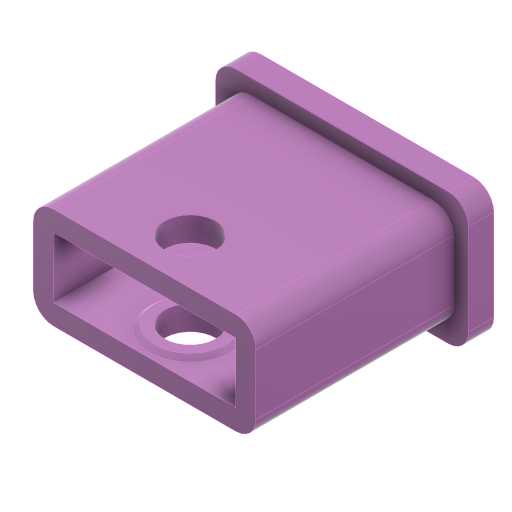
# Autodesk Inventor part: Короб для подшипника
Saved by Autodesk Inventor 2023 (Build 270158000, 158)
## iProperties
Created: 2023-02-25
Part Number: Короб для подшипника
Material: Типовые
Document SubType Name: Modeling
Designer: Admin
Density: 1 g/cm^3
Appearance: По умолчанию
Author: Admin
Autodesk Inventor part; units mm, degrees
ref_plane "YZ Plane" through (0, 0, 0) normal (1, 0, 0) x (0, 1, 0)
ref_plane "XZ Plane" through (0, 0, 0) normal (0, 1, 0) x (-1, 0, 0)
ref_plane "XY Plane" through (0, 0, 0) normal (0, 0, 1) x (1, 0, 0)
sketch "Эскиз1" plane through (0, 0, 0) normal (0, 0, 1) x (1, 0, 0)
  line L0 (-9, -5) -> (9, -5)
  line L1 (11, -3) -> (11, 3)
  line L2 (9, 5) -> (-9, 5)
  line L3 (-11, 3) -> (-11, -3)
  line L4 (-11, -5) -> (11, 5) construction
  line L5 (11, -5) -> (-11, 5) construction
  arc A0 (-9, 5) -> (-11, 3) centre (-9, 3) ccw
  arc A1 (-11, -3) -> (-9, -5) centre (-9, -3) ccw
  arc A2 (9, -5) -> (11, -3) centre (9, -3) ccw
  arc A3 (11, 3) -> (9, 5) centre (9, 3) ccw
  line L6 (-10.5, 6.5) -> (10.5, 6.5)
  line L7 (12.5, 4.5) -> (12.5, -4.5)
  line L8 (10.5, -6.5) -> (-10.5, -6.5)
  line L9 (-12.5, -4.5) -> (-12.5, 4.5)
  line L10 (-12.5, 6.5) -> (12.5, -6.5) construction
  line L11 (12.5, 6.5) -> (-12.5, -6.5) construction
  arc A4 (-10.5, 6.5) -> (-12.5, 4.5) centre (-10.5, 4.5) ccw
  arc A5 (-12.5, -4.5) -> (-10.5, -6.5) centre (-10.5, -4.5) ccw
  arc A6 (10.5, -6.5) -> (12.5, -4.5) centre (10.5, -4.5) ccw
  arc A7 (12.5, 4.5) -> (10.5, 6.5) centre (10.5, 4.5) ccw
  line L12 (-9, -3) -> (9, -3)
  line L13 (9, -3) -> (9, 3)
  line L14 (9, 3) -> (-9, 3)
  line L15 (-9, 3) -> (-9, -3)
  line L16 (-9, -3) -> (9, 3) construction
  line L17 (9, -3) -> (-9, 3) construction
  line L18 (0, 0) -> (7.9203, 0) construction
  dimension "Down_fit_y" = 10
  dimension "Down_fit_x" = 22
  dimension "d2" = 2
  dimension "Up_fit" = 1.5
  dimension "d4" = 1.5
  dimension "d5" = 2
  constraints: 38 end point, 16 point on circle, 16 point on line, 16 tangent, 8 centre point, 7 parallel, 6 equal radius, 6 midpoint, 3 horizontal, 3 perpendicular
  measures "Down_fit_y" distance between parallel lines of L0 L2
  measures "Down_fit_x" distance between parallel lines of L3 L1
  measures "d2" radius of A0
  measures "Up_fit" distance between parallel lines of L6 L2
  measures "d4" distance between parallel lines of L7 L1
  measures "d5" radius of A4
extrude "Выдавливание1" add sketch "Эскиз1" against normal blind 2.5 contours A1 L3 A0 L2 A3 L1 A2 L0 | L6 A7 L7 A6 L8 A5 L9 A4 | L15 L14 L13 L12
extrude "Выдавливание2" add sketch "Эскиз1" along normal blind 19.5 contours A1 L3 A0 L2 A3 L1 A2 L0
sketch "Эскиз2" plane through (-9, 5, 0) normal (0, 1, 0) x (1, 0, 0)
  circle A0 centre (9, -15) radius 2.5
  line L0 (6.6906, -11) -> (11.3094, -11)
  line L1 (11.3094, -11) -> (13.6188, -15)
  line L2 (13.6188, -15) -> (11.3094, -19)
  line L3 (11.3094, -19) -> (6.6906, -19)
  line L4 (6.6906, -19) -> (4.3812, -15)
  line L5 (4.3812, -15) -> (6.6906, -11)
  line L6 (-1.5, 2.5) -> (19.5, 2.5) projected
  line L7 (-2, 0) -> (-2, -19.5) projected
  line L8 (-2, -7.5) -> (20, -7.5) construction
  line L9 (20, 0) -> (20, -19.5) projected
  line L10 (19.5, 0) -> (-1.5, 0) projected
  circle A1 centre (9, -15) radius 8 construction
  line L11 (18, -19.5) -> (0, -19.5) projected
  point P0 (9, 0)
  point P1 (9, 0)
  dimension "hole" = 5
  dimension "d13" = 10
  dimension "d14" = 8
  dimension "d15" = 16
  dimension "d16" = 3.5
  constraints: 14 end point, 2 centre point, 2 coincident, 2 horizontal, 2 point on line, 1 midpoint, 1 vertical alignment, 13 other
  measures "hole" diameter of A0
  measures "d13" distance between parallel lines of L6 L8
  measures "d14" distance between parallel lines of L3 L0
  measures "d15" diameter of A1
  measures "d16" distance edge to line of A1 L11
extrude "Выдавливание3" cut sketch "Эскиз2" against normal through all contours A0
sketch "Эскиз3" plane through (-9, 3, 0) normal (0, -1, 0) x (1, 0, 0)
  circle A0 centre (9, 15) radius 2.5 projected
  circle A1 centre (9, 15) radius 4
  point P0 (9, 0)
  dimension "d19" = 8
  constraints: 1 centre point, 1 coincident
  measures "d19" diameter of A1
extrude "Выдавливание4" add sketch "Эскиз3" along normal blind 0.4
chamfer "Фаска1" distance 0.5 distance2 0.4 1 edges at (-4, 2.6, 15) measured on face at (-3.5, 2.6, 15)
ref_plane "РабПлоскость1" through (0, 0, 0) normal (0, -1, 0) x (1, 0, 0)
mirror "Зеркальное отражение1" about plane through (0, 0, 0) normal (0, -1, 0) of "Выдавливание4", "Фаска1"
equation "\"d4\" = Up_fit"
